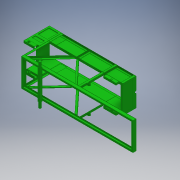
# Autodesk Inventor part: MAIN FRAME
Saved by Autodesk Inventor 2017 (Build 210142000, 142)
## iProperties
Created: 2017-04-14
Part Number: MAIN FRAME
Material: Generic
Document SubType Name: Modeling
Designer: master
Density: 1 g/cm^3
Appearance: Dark Green
Mass: 4.49609 g
Surface Area: 246.253 cm^2
Volume: 4.49609 cm^3
Author: master
Autodesk Inventor part; units mm, degrees
ref_plane "YZ Plane" through (0, 0, 0) normal (1, 0, 0) x (0, 1, 0)
ref_plane "XZ Plane" through (0, 0, 0) normal (0, 1, 0) x (-1, 0, 0)
sketch "Sketch2" plane through (0, 0, 0) normal (1, 0, 0) x (0, 1, 0)
  line L0 (0, 0) -> (0, -1.8819)
  line L1 (0, 0) -> (4, 0)
  line L2 (4, 0) -> (4, -1.8819)
  line L3 (0.236, -1.8891) -> (0.236, -0.236)
  line L4 (0.236, -0.236) -> (3.7638, -0.236)
  line L5 (3.7638, -0.236) -> (3.7638, -1.8819)
  arc A0 (3.7638, -1.8819) -> (4, -1.8819) centre (3.8819, -1.8819) ccw
  line L6 (2, 0) -> (2, -1.818) construction
  arc A1 (0, -1.8819) -> (0.2362, -1.8819) centre (0.1181, -1.8819) ccw
  dimension "d1" = 4
  dimension "d6" = 2
  dimension "d7" = 0.1181
  dimension "d8" = 0.236
  dimension "d9" = 0.236
  constraints: 14 end point, 5 point on circle, 4 perpendicular, 3 symmetric about line, 2 centre point, 2 tangent, 2 vertical, 1 midpoint, 1 parallel, 1 other
  measures "d1" distance of L0.start L1.end
  measures "d7" radius of A1
  measures "d8" distance between parallel lines of L0 L3
  measures "d9" distance between parallel lines of L4 L1
extrude "Extrusion1" add sketch "Sketch2" along normal blind 144
ref_plane "Work Plane1" through (0, 0, -18) normal (0, 0, 1) x (1, 0, 0)
mirror "Mirror1" about plane through (0, 0, -18) normal (0, 0, 1) of "Extrusion1"
sketch "Sketch3" plane through (0, 0, 0) normal (0, 0, 1) x (1, 0, 0)
  line L0 (0, 0) -> (1.8819, 0)
  line L1 (0, 0) -> (0, 4)
  line L2 (0, 4) -> (1.8819, 4)
  line L3 (1.8891, 0.236) -> (0.236, 0.236)
  line L4 (0.236, 0.236) -> (0.236, 3.7638)
  line L5 (0.236, 3.7638) -> (1.8819, 3.7638)
  arc A0 (1.8819, 3.7638) -> (1.8819, 4) centre (1.8819, 3.8819) ccw
  line L6 (0, 2) -> (1.818, 2) construction
  arc A1 (1.8819, 0) -> (1.8819, 0.2362) centre (1.8819, 0.1181) ccw
  dimension "d18" = 2
  dimension "d19" = 4
  dimension "d20" = 0.236
  dimension "d21" = 0.1181
  dimension "d22" = 0.236
  constraints: 14 end point, 5 point on circle, 4 perpendicular, 3 symmetric about line, 2 centre point, 2 tangent, 1 midpoint, 1 parallel, 1 other
  measures "d19" distance between parallel lines of L2 L0
  measures "d20" distance between parallel lines of L4 L1
  measures "d21" radius of A1
  measures "d22" distance between parallel lines of L3 L0
extrude "Extrusion2" add sketch "Sketch3" against normal blind 36
ref_plane "Work Plane2" through (72, 0, 0) normal (-1, 0, 0) x (0, 0, 1)
mirror "Mirror2" about plane through (72, 0, 0) normal (-1, 0, 0) of "Extrusion2"
sketch "Sketch4" plane through (0, 4, 0) normal (0, 1, 0) x (1, 0, 0)
  line L0 (0, 0) -> (2.382, 0)
  line L1 (0, 0) -> (144, 0) projected
  line L2 (0, 0) -> (0, 2.382)
  line L3 (0, 0) -> (0, 36) projected
  line L4 (0, 0) -> (2.618, 0) construction
  line L5 (0.236, 2.382) -> (0.236, 0.236)
  line L6 (0.236, 0.236) -> (2.382, 0.236)
  arc A0 (0.236, 2.382) -> (0, 2.382) centre (0.118, 2.382) ccw
  arc A1 (2.382, 0) -> (2.382, 0.236) centre (2.382, 0.118) ccw
  line L7 (0, 18) -> (26.277, 18) construction
  line L8 (0, 36) -> (2.382, 36)
  line L9 (0, 36) -> (0, 33.618)
  line L10 (0, 36) -> (2.618, 36) construction
  line L11 (0.236, 33.618) -> (0.236, 35.764)
  line L12 (0.236, 35.764) -> (2.382, 35.764)
  arc A2 (0, 33.618) -> (0.236, 33.618) centre (0.118, 33.618) ccw
  arc A3 (2.382, 35.764) -> (2.382, 36) centre (2.382, 35.882) ccw
  line L13 (36, 27.0214) -> (36, 11.3013) construction
  line L14 (72, 0) -> (69.618, 0)
  line L15 (72, 0) -> (72, 2.382)
  line L16 (72, 0) -> (69.382, 0) construction
  line L17 (71.764, 2.382) -> (71.764, 0.236)
  line L18 (71.764, 0.236) -> (69.618, 0.236)
  arc A4 (72, 2.382) -> (71.764, 2.382) centre (71.882, 2.382) ccw
  arc A5 (69.618, 0.236) -> (69.618, 0) centre (69.618, 0.118) ccw
  line L19 (72, 36) -> (69.618, 36)
  line L20 (72, 36) -> (72, 33.618)
  line L21 (72, 36) -> (69.382, 36) construction
  line L22 (71.764, 33.618) -> (71.764, 35.764)
  line L23 (71.764, 35.764) -> (69.618, 35.764)
  arc A6 (71.764, 33.618) -> (72, 33.618) centre (71.882, 33.618) ccw
  arc A7 (69.618, 36) -> (69.618, 35.764) centre (69.618, 35.882) ccw
  dimension "d28" = 90
  dimension "d30" = 0.236
  dimension "d31" = 2.5
  dimension "d34" = 0.118
  dimension "d36" = 2.5
  dimension "d37" = 36
  constraints: 44 end point, 26 symmetric about line, 16 point on circle, 8 centre point, 5 point on line, 4 tangent, 2 horizontal, 1 collinear, 1 midpoint, 1 parallel, 1 perpendicular, 1 vertical, 6 other
  measures "d28" angle of L4 L2
  measures "d30" distance between parallel lines of L0 L6
  measures "d34" radius of A0
  measures "d37" distance between parallel lines of L13 L3
extrude "Extrusion3" add sketch "Sketch4" along normal blind 48
sketch "Sketch6" plane through (0, 0, 0) normal (-1, 0, 0) x (0, 0, 1)
  arc A0 (-0.118, 51.764) -> (-0.118, 52) centre (-0.118, 51.882) ccw
  line L0 (-0.118, 51.764) -> (-2.264, 51.764)
  arc A1 (-2.5, 49.618) -> (-2.264, 49.618) centre (-2.382, 49.618) ccw
  line L1 (-2.5, 52) -> (-0.118, 52)
  line L2 (-2.5, 52) -> (-2.5, 49.618)
  line L3 (-2.5, 52) -> (-2.5, 49.382) construction
  line L4 (-2.264, 51.764) -> (-2.264, 49.618)
  line L5 (-2.5, 4) -> (-2.5, 52) projected
  line L6 (-2.382, 52) -> (0, 52) projected
  line L7 (-2.382, 52) -> (-2.5, 52) projected
  line L8 (0, 0) -> (0, 52) projected
  line L9 (0, 0) -> (-36, 0) projected
  dimension "d43" = 52
  dimension "d44" = 0.236
  dimension "d45" = 0.118
  dimension "d46" = 2.382
  dimension "d47" = 0.236
  dimension "d49" = 2.146
  dimension "d50" = 2.382
  constraints: 10 end point, 4 point on circle, 2 centre point, 1 point on line
  measures "d43" distance between parallel lines of L9 L1
  measures "d44" distance between parallel lines of L1 L0
  measures "d45" radius of A0
  measures "d46" distance from line of L3 A0.centre
  measures "d47" distance between parallel lines of L4 L3
  measures "d49" distance of L0.end L4.end
  measures "d50" distance from line of L1 A1.centre
extrude "Extrusion5" add sketch "Sketch6" against normal blind 96 contours L0 L4 A1 L2 L1 A0
ref_plane "Work Plane4" through (0, 0, -18) normal (0, 0, 1) x (1, 0, 0)
mirror "Mirror3" about plane through (0, 0, -18) normal (0, 0, 1) of "Extrusion5"
ref_plane "Work Plane5" through (48, 0, 0) normal (-1, 0, 0) x (0, 0, 1)
sketch "Sketch8" plane through (0, 0, 0) normal (-1, 0, 0) x (0, 0, 1)
  line L0 (-2.5, 51.7629) -> (-33.5, 51.7629) construction
  line L1 (-2.5, 51.7629) -> (-2.382, 34.7633) construction
  line L2 (-2.382, 4) -> (-2.382, 49.5) construction
  line L3 (-2.382, 34.7633) -> (0, 34.7633)
  arc A0 (-2.146, 37.1453) -> (-2.382, 37.1453) centre (-2.264, 37.1453) ccw
  line L4 (-2.146, 34.9993) -> (0, 34.9993)
  line L5 (-2.382, 34.7633) -> (-2.382, 37.1453)
  line L6 (-2.382, 34.7633) -> (0.236, 34.7633) construction
  arc A1 (0, 34.7633) -> (0, 34.9993) centre (0, 34.8813) ccw
  line L7 (-2.146, 37.1453) -> (-2.146, 34.9993)
  point P0 (0, 0)
  dimension "d62" = 17
  dimension "d63" = 90
  dimension "d64" = 0.236
  dimension "d65" = 2.5
  dimension "d66" = 0.118
  dimension "d67" = 2.5
  constraints: 12 end point, 4 point on circle, 4 tangent, 2 centre point, 2 point on line, 1 parallel, 1 perpendicular
  measures "d62" distance of L0.start L1.end
  measures "d63" angle of L6 L5
  measures "d64" distance between parallel lines of L3 L4
  measures "d66" radius of A0
extrude "Extrusion7" add sketch "Sketch8" against normal blind 96
mirror "Mirror5" about plane through (0, 0, -18) normal (0, 0, 1) of "Extrusion7"
sketch "Sketch10" plane through (72, 34.9993, -33.854) normal (0, 1, 0) x (1, 0, 0)
  line L0 (24, -0.354) -> (24, 2.028) projected
  line L1 (0, 2.028) -> (24, 2.028) projected
  line L2 (24, 2.146) -> (0, 2.146) projected
  line L3 (24, 2.146) -> (24, 2.028) projected
  line L4 (-72, 2.146) -> (-72, -0.354) projected
  line L5 (-72, -0.354) -> (24, -0.354) projected
  line L6 (24, -0.354) -> (24, 2.028) projected
  line L7 (0, 2.028) -> (24, 2.028) projected
  line L8 (0, 2.028) -> (0, 2.146) projected
  line L9 (0, 2.146) -> (-2.382, 2.146) projected
  arc A0 (-2.382, 2.146) -> (-2.5, 2.028) centre (-2.382, 2.028) ccw projected
  line L10 (-69.5, 2.028) -> (-2.5, 2.028) projected
  arc A1 (-69.5, 2.028) -> (-69.618, 2.146) centre (-69.618, 2.028) ccw projected
  line L11 (-69.618, 2.146) -> (-72, 2.146) projected
  line L12 (24, 2.146) -> (21.618, 2.146)
  arc A2 (23.764, -0.236) -> (24, -0.236) centre (23.882, -0.236) ccw
  line L13 (23.764, 1.91) -> (21.618, 1.91)
  line L14 (24, 2.146) -> (24, -0.236)
  line L15 (24, 2.146) -> (21.382, 2.146) construction
  arc A3 (21.618, 2.146) -> (21.618, 1.91) centre (21.618, 2.028) ccw
  line L16 (23.764, -0.236) -> (23.764, 1.91)
  point P0 (-72, -33.854)
  point P1 (24, 2.146)
  dimension "d71" = 90
  dimension "d72" = 0.236
  dimension "d73" = 2.5
  dimension "d74" = 0.118
  dimension "d75" = 2.5
  constraints: 10 end point, 4 point on circle, 4 tangent, 2 centre point, 1 parallel, 1 perpendicular, 1 point on line
  measures "d71" angle of L15 L14
  measures "d72" distance between parallel lines of L12 L13
  measures "d74" radius of A2
extrude "Extrusion8" add sketch "Sketch10" along normal blind 16.8 contours A2 L16 L13 A3 L1 L0 | L1 A3 L2 L3
mirror "Mirror6" about plane through (0, 0, -18) normal (0, 0, 1) of "Extrusion8"
sketch "Sketch11" plane through (96, 34.7633, -2.382) normal (0, 0, -1) x (-1, 0, 0)
  line L0 (0, 0) -> (2.382, 0)
  arc A0 (0.236, 2.382) -> (0, 2.382) centre (0.118, 2.382) ccw
  line L1 (0.236, 0.236) -> (2.382, 0.236)
  line L2 (0, 0) -> (0, 2.382)
  line L3 (0, 0) -> (2.618, 0) construction
  arc A1 (2.382, 0) -> (2.382, 0.236) centre (2.382, 0.118) ccw
  line L4 (0.236, 2.382) -> (0.236, 0.236)
  line L5 (24, 2.382) -> (0.236, 2.382) projected
  line L6 (0.236, 2.5) -> (24, 2.5) projected
  line L7 (2.5, 0.236) -> (2.5, 17.0007) projected
  line L8 (0, 0.236) -> (0, 0) projected
  line L9 (24, 0) -> (0, 0) projected
  point P0 (96, -34.7633)
  point P1 (0, 0)
  dimension "d78" = 90
  dimension "d79" = 0.236
  dimension "d80" = 2.5
  dimension "d81" = 0.118
  dimension "d82" = 2.5
  constraints: 10 end point, 4 point on circle, 4 tangent, 2 centre point, 1 parallel, 1 perpendicular, 1 point on line
  measures "d78" angle of L3 L2
  measures "d79" distance between parallel lines of L0 L1
  measures "d81" radius of A0
extrude "Extrusion9" add sketch "Sketch11" against normal up to surface (31.236 mm away) from surface at 31.236
ref_plane "Work Plane8" through (0, 0, 0) normal (0.6819984, 0.7313537, 0) x (0, 0, -1)
sketch "Sketch12" plane through (0, 0, 0) normal (0.6819984, 0.7313537, 0) x (0, 0, -1)
  arc A0 (35.9998, -0.4142) -> (35.9998, -0.1782) centre (35.9998, -0.2962) ccw
  line L0 (35.9998, -0.4142) -> (33.8538, -0.4142)
  arc A1 (33.6178, -2.5602) -> (33.8538, -2.5602) centre (33.7358, -2.5602) ccw
  line L1 (33.6178, -0.1782) -> (35.9998, -0.1782)
  line L2 (33.6178, -0.1782) -> (33.6178, -2.5602)
  line L3 (33.6178, -0.1782) -> (33.6178, -2.7962) construction
  line L4 (33.8538, -0.4142) -> (33.8538, -2.5602)
  line L5 (36.118, -46.421) -> (36.118, 23.789) projected
  point P0 (0, 0)
  constraints: 10 end point, 4 point on circle, 2 centre point, 1 point on line
extrude "Extrusion10" add sketch "Sketch12" along normal up to surface starts on plane at (0, 4, -1.8819) facing (0, 1, 0) surface through (0, 34.7633, 0) normal (0, -1, 0)
ref_plane "Work Plane9" through (36.118, 4, -33.618) normal (1, 0, 0) x (0, 0, -1)
mirror "Mirror7" about plane through (36.118, 4, -33.618) normal (1, 0, 0) of "Extrusion10"
mirror "Mirror8" about plane through (0, 0, -18) normal (0, 0, 1) of "Extrusion10", "Mirror7"
sketch "Sketch14" plane through (0.236, 34.9993, -33.854) normal (0, 1, 0) x (1, 0, 0)
  line L0 (-0.236, -33.854) -> (-0.236, 2.146) construction
  line L1 (-0.236, -0.7065) -> (35.7571, 0) construction
  line L2 (0, 0) -> (71.528, 0) construction
  line L3 (35.7571, 0) -> (40.4608, -19.6058) construction
  line L4 (35.8446, -0.3454) -> (38.2266, -0.3454)
  arc A0 (36.0806, 2.0366) -> (35.8446, 2.0366) centre (35.9626, 2.0366) ccw
  line L5 (36.0806, -0.1094) -> (38.2266, -0.1094)
  line L6 (35.8446, -0.3454) -> (35.8446, 2.0366)
  line L7 (35.8446, -0.3454) -> (38.4626, -0.3454) construction
  arc A1 (38.2266, -0.3454) -> (38.2266, -0.1094) centre (38.2266, -0.2274) ccw
  line L8 (36.0806, 2.0366) -> (36.0806, -0.1094)
  line L9 (35.8446, -0.1094) -> (35.8446, -0.3454)
  point P0 (35.8446, -0.3454)
  point P1 (36.0806, 2.0366)
  point P2 (36.0806, 2.1546)
  point P3 (38.3446, -0.1094)
  dimension "d89" = 36
  dimension "d90" = 90
  dimension "d91" = 0.236
  dimension "d92" = 2.5
  dimension "d93" = 0.118
  dimension "d94" = 2.5
  constraints: 16 end point, 4 point on circle, 4 tangent, 3 point on line, 2 centre point, 1 parallel, 1 perpendicular
  measures "d89" distance of L1.start L1.end
  measures "d90" angle of L7 L6
  measures "d91" distance between parallel lines of L4 L5
  measures "d93" radius of A0
extrude "Extrusion11" add sketch "Sketch14" along normal up to surface (16.7647 mm away) from surface at 0
mirror "Mirror9" about plane through (0, 0, -18) normal (0, 0, 1) of "Extrusion11"
sketch "Sketch17" plane through (0, 52, -33.5) normal (0, 0, 1) x (1, 0, 0)
  line L0 (0.236, -0.2371) -> (2.382, -0.2371) projected
  line L1 (96, -17.0007) -> (96, -17.2367) projected
  line L2 (0.236, -0.2371) -> (96, -0.2371)
  line L3 (96, -0.2371) -> (96, -17.2367)
  line L4 (96, -17.2367) -> (0.236, -17.2367)
  line L5 (0.236, -17.2367) -> (0.236, -0.2371)
  point P0 (0, -52)
  constraints: 8 end point, 2 parallel, 1 horizontal, 1 perpendicular
extrude "Extrusion13" add sketch "Sketch17" against normal blind 0.1
mirror "Mirror10" about plane through (0, 0, -18) normal (0, 0, 1) of "Extrusion13"
ref_plane "Work Plane10" through (72, 41.2633, 0) normal (0, -1, 0) x (1, 0, 0)
mirror "Mirror11" about plane through (72, 41.2633, 0) normal (0, -1, 0) of "Extrusion9"
sketch "Sketch18" plane through (96, 0, 0) normal (1, 0, 0) x (0, 0, -1)
  line L0 (0.118, 52) -> (0, 52) projected
  line L1 (36, 4) -> (36, 34.7633) projected
  line L2 (0, 52) -> (36, 52)
  line L3 (36, 52) -> (36, 34.7633)
  line L4 (36, 34.7633) -> (0, 34.7633)
  line L5 (0, 34.7633) -> (0, 52)
  point P0 (0, 0)
  constraints: 8 end point, 2 parallel, 1 horizontal, 1 perpendicular
extrude "Extrusion14" add sketch "Sketch18" against normal blind 0.24
mirror "Mirror12" about plane through (48, 0, 0) normal (-1, 0, 0) of "Extrusion9", "Mirror11", "Extrusion14"
sketch "Sketch19" plane through (0, 0, 0) normal (-1, 0, 0) x (0, 0, 1)
  line L0 (-36, 52) -> (0, 52) projected
  circle A0 centre (-18, 52) radius 1.5
  point P0 (0, 0)
  dimension "d104" = 3
  constraints: 1 centre point, 1 midpoint
  measures "d104" diameter of A0
extrude "Extrusion15" cut sketch "Sketch19" against normal blind 114 and the other way blind 67
sketch "Sketch21" plane through (72, 34.7633, 0) normal (0, -1, 0) x (1, 0, 0)
  line L0 (24, -36.118) -> (-72, -36.118) projected
  line L1 (3.1715, -36.118) -> (19.3506, -36.118)
  line L2 (19.3506, -36.118) -> (19.3506, -35.878)
  line L3 (19.3506, -35.878) -> (3.1715, -35.878)
  line L4 (3.1715, -35.878) -> (3.1715, -36.118)
  point P0 (-72, 0)
  dimension "d111" = 0.24
  constraints: 8 end point, 2 parallel, 1 horizontal, 1 perpendicular, 1 point on line
  measures "d111" distance of L2.end L1.end
extrude "Extrusion17" add sketch "Sketch21" along normal blind 4
sketch "Sketch22" plane through (72, 30.7633, 0) normal (0, -1, 0) x (1, 0, 0)
  line L0 (3.1715, -36.118) -> (19.3506, -36.118) projected
  line L1 (0, -33.736) -> (23.76, -33.736) projected
  line L2 (3.1715, -36.118) -> (19.353, -36.118)
  line L3 (19.353, -36.118) -> (19.353, -33.736)
  line L4 (19.353, -33.736) -> (3.1715, -33.736)
  line L5 (3.1715, -33.736) -> (3.1715, -36.118)
  point P0 (-72, 0)
  constraints: 8 end point, 2 parallel, 1 horizontal, 1 perpendicular, 1 point on line
extrude "Extrusion18" add sketch "Sketch22" against normal blind 0.24
sketch "Sketch23" plane through (91.353, 30.7633, -33.736) normal (1, 0, 0) x (0, 0, -1)
  line L0 (0, 0) -> (0, 0.24) projected
  line L1 (2.3818, 4) -> (2.3818, -26.7633) projected
  line L2 (0, 0) -> (2.3818, 0)
  line L3 (2.3818, 0) -> (2.3818, 4)
  line L4 (2.3818, 4) -> (0, 4)
  line L5 (0, 4) -> (0, 0)
  point P0 (-33.736, -30.7633)
  constraints: 8 end point, 2 parallel, 1 horizontal, 1 perpendicular, 1 point on line
extrude "Extrusion19" add sketch "Sketch23" against normal blind 0.24
sketch "Sketch24" plane through (75.1715, 30.7633, -36.118) normal (-1, 0, 0) x (0, 0, 1)
  line L0 (0, 0) -> (0, 0.24) projected
  line L1 (2.382, 4) -> (0.118, 4) projected
  line L2 (0, 0) -> (2.382, 0)
  line L3 (2.382, 0) -> (2.382, 4)
  line L4 (2.382, 4) -> (0, 4)
  line L5 (0, 4) -> (0, 0)
  point P0 (36.118, -30.7633)
  constraints: 8 end point, 2 parallel, 1 horizontal, 1 perpendicular
extrude "Extrusion20" add sketch "Sketch24" against normal blind 0.24
sketch "Sketch25" plane through (91.113, 31.0033, -35.878) normal (0, 0, 1) x (1, 0, 0)
  circle A0 centre (-7.0341, 1.3535) radius 0.75
  circle A1 centre (-7.0341, 1.3535) radius 1.3535
  line L0 (-15.7015, 0) -> (0, 0) projected
  point P0 (-91.113, -31.0033)
  dimension "d120" = 1.5
  constraints: 2 centre point, 1 coincident, 1 tangent
  measures "d120" diameter of A0
extrude "Extrusion21" add sketch "Sketch25" along normal blind 1.5
mirror "Mirror13" about plane through (0, 0, -18) normal (0, 0, 1) of "Extrusion21", "Extrusion18", "Extrusion20", "Extrusion17", "Extrusion19"
sketch "Sketch26" plane through (75.1715, 30.7633, 0.118) normal (0, 0, 1) x (1, 0, 0)
  circle A0 centre (8.9074, 1.5935) radius 0.75 projected
  line L0 (8.9074, 1.5935) -> (-86.6339, -10.0069) construction
  line L1 (8.9074, 1.5935) -> (105.1504, 1.5935) construction
  circle A1 centre (-86.6339, -10.0069) radius 1
  circle A2 centre (-86.6339, -10.0069) radius 1.75
  line L2 (-91.0537, -11.7569) -> (-77.2677, -11.7569)
  line L3 (-74.9355, -26.7633) -> (-74.9355, 4) projected
  line L4 (-77.2677, -11.7569) -> (-77.2677, -7.6624)
  line L5 (-77.2677, -7.6624) -> (-91.0537, -7.6624)
  line L6 (-91.0537, -7.6624) -> (-91.0537, -11.7569)
  point P0 (-75.1715, -30.7633)
  dimension "d123" = 96.243
  dimension "d125" = 2
  dimension "d126" = 3.5
  dimension "d173" = 4.0945
  dimension "d174" = 13.786
  constraints: 12 end point, 4 perpendicular, 2 centre point, 2 coincident, 1 equal length, 1 horizontal, 1 tangent
  measures "d123" distance of L0.start L0.end
  measures "d125" diameter of A1
  measures "d126" diameter of A2
  measures "d173" distance of L5.end L2.start
  measures "d174" distance between parallel lines of L4 L6
extrude "Extrusion22" add sketch "Sketch26" along normal up to surface (2.3822 mm away) from surface at -2.5002 contours A2
extrude "Extrusion23" add sketch "Sketch26" against normal blind 0.24 contours L2 L6 L5 L4
sketch "Sketch27" plane through (75.1715, 30.7633, 0.118) normal (0, 0, 1) x (1, 0, 0)
  line L0 (-75.1715, 4.236) -> (-75.1715, 21.2367) projected
  line L1 (-77.2677, -7.6624) -> (-91.0537, -7.6624) projected
  line L2 (-75.1715, 21.2367) -> (-91.0537, 21.2367)
  line L3 (-91.0537, 21.2367) -> (-91.0537, -7.6624)
  line L4 (-91.0537, -7.6624) -> (-75.1715, -7.6624)
  line L5 (-75.1715, -7.6624) -> (-75.1715, 21.2367)
  point P0 (-75.1715, -30.7633)
  constraints: 8 end point, 2 parallel, 1 horizontal, 1 perpendicular
extrude "Extrusion26" add sketch "Sketch27" against normal blind 2.49
sketch "Sketch28" plane through (-15.8823, 19.0064, 0.118) normal (-1, 0, 0) x (0, 0, 1)
  line L0 (-2.5002, -15.0064) -> (-2.5002, 15.7569) projected
  line L1 (-2.5, -15.0064) -> (-2.5, 15.7569) projected
  line L2 (-2.5, 4.2034) -> (-0.24, 4.2034)
  line L3 (-0.24, 4.2034) -> (-0.24, 0)
  line L4 (-0.24, 0) -> (-2.5, 0)
  line L5 (-2.5, 0) -> (-2.5, 4.2034)
  point P0 (-0.118, -19.0064)
  point P1 (-2.5002, 4.0743)
  constraints: 8 end point, 2 parallel, 2 point on line, 1 horizontal, 1 perpendicular
extrude "Extrusion27" add sketch "Sketch28" against normal blind 0.24
sketch "Sketch29" plane through (-11.4624, 19.0064, 0.118) normal (0, -1, 0) x (1, 0, 0)
  line L0 (-4.1798, -2.49) -> (-4.4198, -2.49) projected
  line L1 (0, 0) -> (9.3662, 0) projected
  line L2 (-4.4198, -2.49) -> (9.3662, -2.49)
  line L3 (9.3662, -2.49) -> (9.3662, 0)
  line L4 (9.3662, 0) -> (-4.4198, 0)
  line L5 (-4.4198, 0) -> (-4.4198, -2.49)
  point P0 (11.4624, -0.118)
  constraints: 8 end point, 2 parallel, 1 horizontal, 1 perpendicular
extrude "Extrusion28" add sketch "Sketch29" along normal blind 0.24
sketch "Sketch30" plane through (75.1715, 30.7633, 0.118) normal (0, 0, 1) x (1, 0, 0)
  line L0 (-89.1355, 18.833) -> (-77.2179, 18.833)
  line L1 (-77.2179, 18.833) -> (-77.2179, 4.6282)
  line L2 (-77.2179, 4.6282) -> (-89.1355, 4.6282)
  line L3 (-89.1355, 4.6282) -> (-89.1355, 18.833)
  point P0 (-75.1715, -30.7633)
  constraints: 8 end point, 2 parallel, 1 horizontal, 1 perpendicular
extrude "Extrusion29" cut sketch "Sketch30" against normal blind 0.7
sketch "Sketch31" plane through (75.1715, 30.7633, 0.118) normal (0, 0, 1) x (1, 0, 0)
  line L0 (-89.1355, 1.225) -> (-77.2179, 1.225)
  line L1 (-77.2179, 1.225) -> (-77.2179, -3.137)
  line L2 (-77.2179, -3.137) -> (-89.1355, -3.137)
  line L3 (-89.1355, -3.137) -> (-89.1355, 1.225)
  point P0 (-75.1715, -30.7633)
  constraints: 8 end point, 2 parallel, 1 horizontal, 1 perpendicular
extrude "Extrusion30" cut sketch "Sketch31" against normal blind 0.7
mirror "Mirror14" about plane through (0, 0, -18) normal (0, 0, 1) of "Extrusion26", "Extrusion29", "Extrusion30", "Extrusion22", "Extrusion23", "Extrusion27", "Extrusion28"
sketch "Sketch32" plane through (0, 0, 0) normal (-1, 0, 0) x (0, 0, 1)
  line L0 (-2.372, 23.2099) -> (-2.372, 52) projected
  line L1 (0.118, 52) -> (-2.372, 52) projected
  line L2 (-2.382, 4) -> (-2.382, 34.7633) projected
  line L3 (-2.382, 4) -> (-33.618, 4) projected
  line L4 (-33.618, 4) -> (-33.618, 34.7633) projected
  line L5 (-33.618, 34.7633) -> (-2.382, 34.7633) projected
  line L6 (-33.628, 52) -> (-33.628, 23.1009) projected
  line L7 (-33.628, 23.1009) -> (-36, 23.1009) projected
  line L8 (-36, 23.1009) -> (-36, 0) projected
  line L9 (0, 0) -> (-36, 0) projected
  line L10 (0, 0) -> (0, 23.1009) projected
  line L11 (0, 23.1009) -> (-2.372, 23.1009) projected
  line L12 (-2.372, 23.1009) -> (-2.372, 52) projected
  line L13 (-16.5, 52) -> (-2.372, 52) projected
  arc A0 (-19.5, 52) -> (-16.5, 52) centre (-18, 52) ccw projected
  line L14 (-33.628, 52) -> (-19.5, 52) projected
  line L15 (-2.372, 52) -> (-33.618, 52)
  line L16 (-33.618, 52) -> (-33.618, 34.7633)
  line L17 (-33.618, 34.7633) -> (-2.372, 34.7633)
  line L18 (-2.372, 34.7633) -> (-2.372, 52)
  constraints: 8 end point, 2 parallel, 1 horizontal, 1 perpendicular
extrude "Extrusion31" cut sketch "Sketch32" against normal blind 7.45 contours L17 L5 L16 L14 A0 L13 L0 | A0 L15
sketch "Sketch33" plane through (-15.8823, 52, -2.372) normal (-1, 0, 0) x (0, 0, 1)
  line L0 (-17.128, 0) -> (-33.628, 0) projected
  line L1 (0.108, -17.2367) -> (2.372, -17.2367) projected
  line L2 (-32.4657, 0) -> (1.24, 0)
  line L3 (1.24, 0) -> (1.24, -17.2367)
  line L4 (1.24, -17.2367) -> (-32.4657, -17.2367)
  line L5 (-32.4657, -17.2367) -> (-32.4657, 0)
  point P0 (2.372, -52)
  constraints: 8 end point, 2 parallel, 1 horizontal, 1 midpoint, 1 perpendicular, 1 point on line
extrude "Extrusion32" add sketch "Sketch33" against normal blind 0.3
sketch "Sketch34" plane through (-15.8823, 19.0064, -2.382) normal (-1, 0, 0) x (0, 0, 1)
  arc A0 (-17.118, 32.9936) -> (-14.118, 32.9936) centre (-15.618, 32.9936) ccw projected
  circle A1 centre (-15.618, 32.9936) radius 1.5
  point P0 (2.382, -19.0064)
  constraints: 1 centre point, 1 coincident
extrude "Extrusion33" cut sketch "Sketch34" against normal blind 6
sketch "Sketch35" plane through (93.618, 34.7633, -2.5) normal (0, 0, -1) x (-1, 0, 0)
  line L0 (86.168, 14.7381) -> (57.5374, 14.7381) projected
  line L1 (93.618, 0.236) -> (93.618, 17.2367) projected
  line L2 (85.6611, 14.7381) -> (93.618, 14.7381)
  line L3 (93.618, 14.7381) -> (93.618, 2.1862)
  line L4 (93.618, 2.1862) -> (85.6611, 2.1862)
  line L5 (85.6611, 2.1862) -> (85.6611, 14.7381)
  point P0 (93.618, -34.7633)
  constraints: 8 end point, 2 parallel, 2 point on line, 1 horizontal, 1 perpendicular
extrude "Extrusion34" add sketch "Sketch35" against normal blind 0.24
sketch "Sketch36" plane through (71.882, 34.7633, -33.5) normal (0, 0, 1) x (1, 0, 0)
  line L0 (-63.992, 15.7828) -> (-72.3184, 15.7828)
  line L1 (-72.3184, 15.7828) -> (-72.3184, 1.9621)
  line L2 (-72.3184, 1.9621) -> (-63.992, 1.9621)
  line L3 (-63.992, 1.9621) -> (-63.992, 15.7828)
  point P0 (-71.882, -34.7633)
  constraints: 8 end point, 2 parallel, 1 horizontal, 1 perpendicular
extrude "Extrusion35" add sketch "Sketch36" against normal blind 0.24
sketch "Sketch37" plane through (0, 0, 0) normal (0, 0, 1) x (1, 0, 0)
  line L0 (1.8819, 0) -> (142.1181, 0) projected
  line L1 (23.9484, 0) -> (26.9484, 0)
  line L2 (26.9484, 0) -> (26.9484, -3)
  line L3 (26.9484, -3) -> (23.9484, -3)
  line L4 (23.9484, -3) -> (23.9484, 0)
  point P0 (0, 0)
  dimension "d158" = 3
  dimension "d159" = 3
  constraints: 8 end point, 2 parallel, 1 horizontal, 1 perpendicular, 1 point on line
  measures "d158" distance of L2.end L3.end
  measures "d159" distance of L1.end L2.end
extrude "Extrusion36" add sketch "Sketch37" along normal blind 1 and the other way blind 37
sketch "Sketch38" plane through (0, 0, 1) normal (0, 0, 1) x (1, 0, 0)
  line L0 (26.9484, -3) -> (26.9484, 0) construction
  line L1 (23.9484, -3) -> (26.9484, -3) construction
  line L2 (23.9484, 0) -> (23.9484, -3) construction
  circle A0 centre (25.4484, -1.5) radius 1.5
  point P0 (0, 0)
  constraints: 3 tangent, 1 centre point
extrude "Extrusion37" add sketch "Sketch38" along normal blind 7 and the other way blind 45
sketch "Sketch39" plane through (144, 4, -36) normal (0, 0, -1) x (-1, 0, 0)
  circle A0 centre (70.5, 10) radius 1
  line L0 (72, 0) -> (72, 30.7633) construction
  line L1 (72, 0) -> (0, 0) projected
  arc A1 (70.5, 11.5) -> (70.5, 8.5) centre (70.5, 10) ccw
  line L2 (70.5, 8.5) -> (72, 8.5)
  line L3 (72, 0) -> (72, 30.7633) projected
  line L4 (72, 11.5) -> (70.5, 11.5)
  line L5 (72, 11.5) -> (72, 8.5)
  point P0 (144, -4)
  dimension "d168" = 2
  dimension "d169" = 10
  dimension "d170" = 3
  constraints: 6 end point, 3 tangent, 2 centre point, 2 perpendicular, 2 point on circle, 2 point on line, 1 coincident
  measures "d168" diameter of A0
  measures "d169" distance from line of A0.centre L1
  measures "d170" diameter of A1
extrude "Extrusion38" add sketch "Sketch39" against normal blind 2.5
mirror "Mirror15" about plane through (0, 0, -18) normal (0, 0, 1) of "Extrusion38"
ref_plane "Work Plane7" through (0, 0, -18) normal (0, 0, 1) x (1, 0, 0)
body "Solid1"
